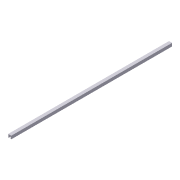
# Autodesk Inventor part: FE-00014-03
Saved by Autodesk Inventor 2012 (Build 160160000, 160)
## iProperties
Company: FIRST
Created: 2008-05-25
Part Number: FE-00014-03
Document SubType Name: Modeling
Designer: dfoster
Density: 1 g/cm^3
Description: Channel
Mass: 159.774 g
Surface Area: 1072.58 cm^2
Volume: 159.774 cm^3
Material: Default
Title: Channel
Author: Dfoster
Autodesk Inventor part; units mm, degrees
ref_plane "YZ Plane" through (0, 0, 0) normal (1, 0, 0) x (0, 1, 0)
ref_plane "XZ Plane" through (0, 0, 0) normal (0, 1, 0) x (-1, 0, 0)
ref_plane "XY Plane" through (0, 0, 0) normal (0, 0, 1) x (1, 0, 0)
sketch "Sketch1" plane through (0, 0, 0) normal (0, 0, 1) x (1, 0, 0)
  line L0 (-22.225, 19.1603) -> (-22.225, 0.1103)
  line L1 (-22.225, 0.1103) -> (-19.05, 0.1103)
  line L2 (-19.05, 0.1103) -> (-19.05, 15.9853)
  line L3 (-19.05, 15.9853) -> (-6.35, 15.9853)
  line L4 (-6.35, 15.9853) -> (-6.35, 0.1103)
  line L5 (-6.35, 0.1103) -> (-3.175, 0.1103)
  line L6 (-3.175, 0.1103) -> (-3.175, 19.1603)
  line L7 (-3.175, 19.1603) -> (-22.225, 19.1603)
  dimension "d0" = 19.05
  dimension "d1" = 19.05
  dimension "d2" = 3.175
  dimension "d3" = 3.175
  constraints: 16 end point, 5 parallel, 2 equal length, 1 collinear, 1 horizontal, 1 vertical
  measures "d0" distance of L6.end L0.start
  measures "d1" distance of L0.start L0.end
  measures "d2" distance between parallel lines of L3 L7
  measures "d3" distance between parallel lines of L2 L0
extrude "Extrusion1" add sketch "Sketch1" along normal blind 990.6
body "Solid1"
